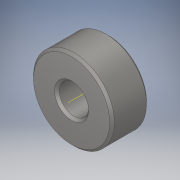
# Autodesk Inventor part: 1603-2RS Ball Bearing 5_16x7_8x11_32 Sealed 1603DC
Saved by Autodesk Inventor 2019.4 (Build 234330000, 330)
## iProperties
Created: 2018-01-08
Part Number: 1603-2RS Ball Bearing 5_16x7_8x11_32 Sealed 1603DC
Material: Steel
Document SubType Name: Modeling
Designer: dlangdon
Density: 7.85 g/cm^3
Appearance: Stainless - Brushed
Mass: 12.7982 g
Surface Area: 9.64933 cm^2
Volume: 1.63034 cm^3
Author: dlangdon
Autodesk Inventor part; units mm, degrees
ref_plane "YZ Plane" through (0, 0, 0) normal (1, 0, 0) x (0, 1, 0)
ref_plane "XZ Plane" through (0, 0, 0) normal (0, 1, 0) x (-1, 0, 0)
ref_plane "XY Plane" through (0, 0, 0) normal (0, 0, 1) x (1, 0, 0)
sketch "Sketch1" plane through (0, 0, 0) normal (0, 0, 1) x (1, 0, 0)
  circle A0 centre (0, 0) radius 3.175
  circle A1 centre (0, 0) radius 8.7313
  dimension "d7" = 6.35
  dimension "d8" = 17.4625
  constraints: 2 centre point, 2 coincident
  measures "d7" diameter of A0
  measures "d8" diameter of A1
extrude "Extrusion1" add sketch "Sketch1" along normal blind 7.9375
chamfer "Chamfer1" distance 0.508 angle 45 4 edges at (-8.7313, 0, 7.9375) (-3.175, 0, 7.9375) (-3.175, 0, 0) (-8.7313, 0, 0)
ref_plane "Work Plane1" through (0, 0, 3.9688) normal (0, 0, 1) x (1, 0, 0)
ref_plane "Work Plane2" through (0, 0, 3.9688) normal (0, 0, 1) x (1, 0, 0)
body "Solid1"
